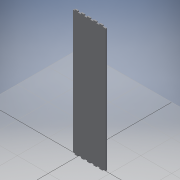
# Autodesk Inventor part: верх
Saved by Autodesk Inventor 2019 (Build 230136000, 136)
## iProperties
Created: 2022-06-29
Part Number: верх
Material: Типовые
Document SubType Name: Modeling
Designer: korsh
Density: 1 g/cm^3
Appearance: По умолчанию
Author: korsh
Autodesk Inventor part; units mm, degrees
ref_plane "YZ Plane" through (0, 0, 0) normal (1, 0, 0) x (0, 1, 0)
ref_plane "XZ Plane" through (0, 0, 0) normal (0, 1, 0) x (-1, 0, 0)
ref_plane "XY Plane" through (0, 0, 0) normal (0, 0, 1) x (1, 0, 0)
sketch "Эскиз1" plane through (0, 0, 0) normal (0, 0, 1) x (1, 0, 0)
  line L0 (-15.776, 404) -> (-10, 404) projected
  line L1 (0, 404) -> (-10, 404) projected
  line L2 (0, 404) -> (0, 408) projected
  line L3 (-10, 408) -> (0, 408) projected
  line L4 (-10, 404) -> (-10, 408) projected
  line L5 (20, 404) -> (10, 404) projected
  line L6 (20, 404) -> (20, 408) projected
  line L7 (10, 408) -> (20, 408) projected
  line L8 (10, 404) -> (10, 408) projected
  line L9 (0, 404) -> (10, 404) projected
  line L10 (20, 404) -> (30, 404) projected
  line L11 (40, 404) -> (30, 404) projected
  line L12 (40, 404) -> (40, 408) projected
  line L13 (30, 408) -> (40, 408) projected
  line L14 (30, 404) -> (30, 408) projected
  line L15 (40, 404) -> (50, 404) projected
  line L16 (60, 404) -> (50, 404) projected
  line L17 (60, 404) -> (60, 408) projected
  line L18 (50, 408) -> (60, 408) projected
  line L19 (50, 404) -> (50, 408) projected
  line L20 (60, 404) -> (70, 404) projected
  line L21 (70, 404) -> (80, 404) projected
  line L22 (80, 404) -> (80, 408) projected
  line L23 (70, 408) -> (80, 408) projected
  line L24 (70, 404) -> (70, 408) projected
  line L25 (80, 404) -> (90.6418, 404) projected
  line L26 (-15.776, 4) -> (-10, 4) projected
  line L27 (0, 0) -> (-10, 0) projected
  line L28 (0, 0) -> (0, 4) projected
  line L29 (-10, 4) -> (0, 4) projected
  line L30 (-10, 0) -> (-10, 4) projected
  line L31 (0, 4) -> (10, 4) projected
  line L32 (20, 0) -> (10, 0) projected
  line L33 (20, 0) -> (20, 4) projected
  line L34 (10, 4) -> (20, 4) projected
  line L35 (10, 0) -> (10, 4) projected
  line L36 (20, 4) -> (30, 4) projected
  line L37 (40, 0) -> (30, 0) projected
  line L38 (40, 0) -> (40, 4) projected
  line L39 (30, 4) -> (40, 4) projected
  line L40 (30, 0) -> (30, 4) projected
  line L41 (60, 0) -> (50, 0) projected
  line L42 (60, 0) -> (60, 4) projected
  line L43 (50, 4) -> (60, 4) projected
  line L44 (50, 0) -> (50, 4) projected
  line L45 (40, 4) -> (50, 4) projected
  line L46 (60, 4) -> (70, 4) projected
  line L47 (70, 0) -> (80, 0) projected
  line L48 (80, 0) -> (80, 4) projected
  line L49 (70, 4) -> (80, 4) projected
  line L50 (70, 0) -> (70, 4) projected
  line L51 (80, 4) -> (90.6418, 4) projected
  line L52 (90.6418, 4) -> (90.6418, 404)
  line L53 (-15.776, 404) -> (-10, 404) projected
  line L54 (-15.776, 4) -> (-15.776, 404)
  constraints: 4 end point, 2 vertical
extrude "Выдавливание1" add sketch "Эскиз1" along normal blind 4
